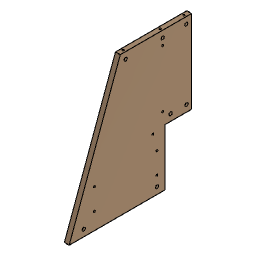
Side Panel Left (Autodesk Fusion 360 design; units mm, degrees)
Autodesk Fusion 360 part; units mm, degrees
note: some values were not read from the file. Set by a fixed rule: which sketch regions a step uses.
sketch "Left" plane through (0, 0, 0) normal (1, 0, 0) x (0, 1, 0)
  line L0 (0, 0) -> (-100, 0) construction
  line L1 (-100, 0) -> (-100, 212.5) construction
  line L2 (-100, 212.5) -> (0, 212.5) construction
  line L3 (0, 212.5) -> (0, 0) construction
  line L4 (0, 212.5) -> (0, 524)
  line L5 (0, 524) -> (-268, 524)
  line L6 (-268, 524) -> (-460, 0)
  line L7 (-460, 0) -> (-100, 0)
  line L8 (-100, 0) -> (-100, 212.5)
  line L9 (-100, 212.5) -> (0, 212.5)
  line L10 (-100, 25) -> (-450.8397, 25) construction
  line L11 (0, 237.5) -> (-372.9771, 237.5) construction
  line L12 (0, 499) -> (-277.1603, 499) construction
  line L13 (-109, 524) -> (-109, 220) construction
  line L14 (-130, 0) -> (-130, 210) construction
  line L15 (-130, 63) -> (-365, 63) construction
  line L16 (-365, 63) -> (-365, 143) construction
  line L17 (-365, 143) -> (-130, 143) construction
  line L18 (-130, 143) -> (-130, 63) construction
  circle A0 centre (-109, 499) radius 6
  circle A1 centre (-248, 499) radius 6
  circle A2 centre (-20, 499) radius 6
  circle A3 centre (-19, 237.5) radius 6
  circle A4 centre (-79, 237.5) radius 6
  circle A5 centre (-130, 25) radius 6
  circle A6 centre (-405, 25) radius 6
  circle A7 centre (-130, 143) radius 3.5
  circle A8 centre (-130, 63) radius 3.5
  circle A9 centre (-365, 63) radius 3.5
  circle A10 centre (-365, 143) radius 3.5
  circle A11 centre (-109, 474) radius 3.5
  circle A12 centre (-109, 259) radius 3.5
  circle A13 centre (-145, 204) radius 3.5
  dimension "d1" = 100
  dimension "d2" = 212.5
  dimension "d3" = 311.5
  dimension "d4" = 268
  dimension "d5" = 360
  dimension "d6" = 25
  dimension "d7" = 25
  dimension "d8" = 25
  dimension "d9" = 109
  dimension "d10" = 30
  dimension "d11" = 235
  dimension "d12" = 80
  dimension "d13" = 63
  dimension "d14" = 12
  dimension "d15" = 12
  dimension "d16" = 12
  dimension "d17" = 12
  dimension "d18" = 12
  dimension "d19" = 12
  dimension "d20" = 12
  dimension "d21" = 7
  dimension "d22" = 7
  dimension "d23" = 7
  dimension "d24" = 7
  dimension "d25" = 7
  dimension "d26" = 7
  dimension "d27" = 7
  dimension "d28" = 60
  dimension "d29" = 19
  dimension "d30" = 89
  dimension "d31" = 139
  dimension "d32" = 25
  dimension "d33" = 215
  dimension "d34" = 55
  dimension "d35" = 36
  dimension "d36" = 275
  constraint horizontal L0
  constraint vertical L1
  constraint horizontal L2
  constraint vertical L3
  constraint coincident L0.start L3.end
  constraint perpendicular L2 L4
  constraint perpendicular L3 L5
  constraint perpendicular L1 L7
  constraint coincident L8 L10.start
  constraint coincident L6 L10.end
  constraint perpendicular L8 L10
  constraint coincident L4 L11.start
  constraint coincident L6 L11.end
  constraint perpendicular L4 L11
  constraint coincident L4 L12.start
  constraint coincident L6 L12.end
  constraint perpendicular L4 L12
  constraint coincident L5 L13.start
  constraint perpendicular L11 L13
  constraint coincident L7 L14.start
  constraint perpendicular L10 L14
  constraint horizontal L15
  constraint vertical L16
  constraint horizontal L17
  constraint vertical L18
  constraint coincident L14 L15.start
  constraint coincident L12 A0.centre
  constraint coincident L13 A0.centre
  constraint coincident L12 A1.centre
  constraint coincident L12 A2.centre
  constraint coincident L11 A3.centre
  constraint coincident L11 A4.centre
  constraint coincident L10 A5.centre
  constraint coincident L14 A5.centre
  constraint coincident L10 A6.centre
  constraint coincident L17.end L18.start
  constraint coincident L15.start L18.end
  constraint coincident L15.end L16.start
  constraint coincident L16.end L17.start
  constraint coincident L13 A11.centre
  constraint coincident L13 A12.centre
  measures "d1" distance of L0.start L0.end
  measures "d2" distance of L0.start L2.end
  measures "d3" distance of L2.end L4.end
  measures "d4" distance of L4.end L5.end
  measures "d5" distance of L0.end L6.end
  measures "d6" distance of L5 L12
  measures "d7" distance of L9 L11
  measures "d8" distance of L7 L10
  measures "d9" distance of L4 L13
  measures "d10" distance of L1 L14
  measures "d11" distance of L15.start L15.end
  measures "d12" distance of L15.start L17.end
  measures "d13" distance of L7 L15
  measures "d14" diameter of A0
  measures "d15" diameter of A1
  measures "d16" diameter of A2
  measures "d17" diameter of A3
  measures "d18" diameter of A4
  measures "d19" diameter of A5
  measures "d20" diameter of A6
  measures "d21" diameter of A7
  measures "d22" diameter of A8
  measures "d23" diameter of A9
  measures "d24" diameter of A10
  measures "d25" diameter of A11
  measures "d26" diameter of A12
  measures "d27" diameter of A13
  measures "d28" distance of A3.centre A4.centre
  measures "d29" distance of L4 A3.centre
  measures "d30" distance of A0.centre A2.centre
  measures "d31" distance of A0.centre A1.centre
  measures "d32" distance of A0.centre A11.centre
  measures "d33" distance of A11.centre A12.centre
  measures "d34" vertical distance of A12.centre A13.centre
  measures "d35" horizontal distance of A12.centre A13.centre
  measures "d36" distance of A5.centre A6.centre
extrude "Extrude1" add sketch "Left" along normal blind 18
sketch "Sketch2" plane through (0, 0, 524) normal (0, 0, 1) x (-1, 0, 0)
  line L0 (0, 0) -> (0, 268)
  line L1 (0, 268) -> (-18, 268)
  line L2 (-18, 268) -> (-18, 0)
  line L3 (-18, 0) -> (0, 0)
  line L4 (-9, 268) -> (-9, 0) construction
  circle A0 centre (-9, 248) radius 3.5
  circle A1 centre (-9, 109) radius 3.5
  circle A2 centre (-9, 20) radius 3.5
  dimension "d39" = 7
  dimension "d40" = 7
  dimension "d41" = 7
  dimension "d42" = 20
  dimension "d43" = 89
  dimension "d44" = 139
  constraint midpoint L1 L4.start
  constraint midpoint L3 L4.end
  constraint coincident L4 A0.centre
  constraint coincident L4 A1.centre
  constraint coincident L4 A2.centre
  measures "d39" diameter of A0
  measures "d40" diameter of A1
  measures "d41" diameter of A2
  measures "d42" distance of L3 A2.centre
  measures "d43" distance of A1.centre A2.centre
  measures "d44" distance of A0.centre A1.centre
extrude "Extrude2" cut sketch "Sketch2" against normal blind 35 contours A0 | A1 | A2
sketch "Sketch3" plane through (0, 0, 212.5) normal (0, 0, -1) x (1, 0, 0)
  line L0 (0, 100) -> (0, 0)
  line L1 (0, 0) -> (18, 0)
  line L2 (18, 0) -> (18, 100)
  line L3 (18, 100) -> (0, 100)
  line L4 (9, 100) -> (9, 0) construction
  circle A0 centre (9, 19) radius 3.5
  circle A1 centre (9, 79) radius 3.5
  dimension "d47" = 7
  dimension "d48" = 7
  dimension "d49" = 19
  dimension "d50" = 60
  constraint midpoint L3 L4.start
  constraint midpoint L1 L4.end
  constraint coincident L4 A0.centre
  constraint coincident L4 A1.centre
  measures "d47" diameter of A0
  measures "d48" diameter of A1
  measures "d49" distance of L1 A0.centre
  measures "d50" distance of A0.centre A1.centre
extrude "Extrude3" cut sketch "Sketch3" against normal blind 35 contours A0 | A1
sketch "Sketch4" plane through (0, 0, 0) normal (0, 0, -1) x (1, 0, 0)
  line L0 (0, 460) -> (0, 100)
  line L1 (0, 100) -> (18, 100)
  line L2 (18, 100) -> (18, 460)
  line L3 (18, 460) -> (0, 460)
  line L4 (9, 100) -> (9, 460) construction
  circle A0 centre (9, 130) radius 3.5
  circle A1 centre (9, 405) radius 3.5
  dimension "d53" = 7
  dimension "d55" = 7
  dimension "d56" = 30
  dimension "d57" = 275
  constraint midpoint L1 L4.start
  constraint midpoint L3 L4.end
  constraint coincident L4 A0.centre
  constraint coincident L4 A1.centre
  measures "d53" diameter of A0
  measures "d55" diameter of A1
  measures "d56" distance of L1 A0.centre
  measures "d57" distance of A0.centre A1.centre
extrude "Extrude4" cut sketch "Sketch4" against normal blind 35 contours A0 | A1
named bodies: "Panel Left"
